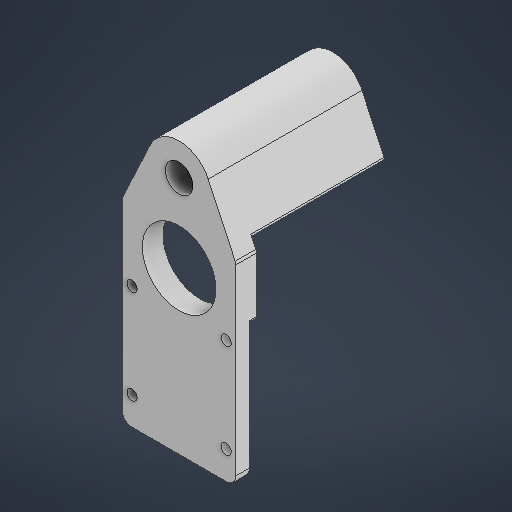
# Autodesk Inventor part: servo_side_plate1
Saved by Autodesk Inventor 2026 (Build 300175000, 175)
## iProperties
Created: 2025-12-05
Part Number: servo_side_plate1
Material: Generic
Document SubType Name: Modeling
Designer: numai
Density: 1 g/cm^3
Appearance: Default
Author: numai
Autodesk Inventor part; units mm, degrees
ref_plane "YZ Plane" through (0, 0, 0) normal (1, 0, 0) x (0, 1, 0)
ref_plane "XZ Plane" through (0, 0, 0) normal (0, 1, 0) x (-1, 0, 0)
ref_plane "XY Plane" through (0, 0, 0) normal (0, 0, 1) x (1, 0, 0)
ref_plane "作業平面1" through (0, -9.51851, 2.5) normal (0, 0, 1) x (1, 0, 0)
sketch "スケッチ1" plane through (0, -9.51851, 2.5) normal (0, 0, 1) x (1, 0, 0)
  arc A0 (6.110987, 12.224368) -> (9.975635, 16.20851) centre (0, 22.01851) ccw construction
  arc A1 (7, 11.230546) -> (6.110987, 12.224368) centre (6, 11.230546) ccw construction
  line L0 (7, 11.230546) -> (7, -12.09149) construction
  arc A2 (6.605696, -12.887186) -> (7, -12.09149) centre (6, -12.09149) ccw construction
  arc A3 (6.605696, -12.887186) -> (7.8, -11.59149) centre (6.5, -11.59149) ccw construction
  line L1 (7.8, -10.59149) -> (7.8, -11.59149) construction
  arc A4 (10.11, -8.28149) -> (7.8, -10.59149) centre (10.11, -10.59149) ccw construction
  line L2 (10.86, -8.28149) -> (10.11, -8.28149) construction
  arc A5 (10.86, -8.28149) -> (12.16, -6.98149) centre (10.86, -6.98149) ccw construction
  line L3 (12.16, 16.20851) -> (12.16, -6.98149) construction
  line L4 (9.975635, 16.20851) -> (12.16, 16.20851) construction
  circle A6 centre (10.25, 13.51851) radius 0.7835 construction
  circle A7 centre (10.25, -6.98149) radius 0.7835 construction
  arc A8 (-7.8, -11.59149) -> (-6.605696, -12.887186) centre (-6.5, -11.59149) ccw construction
  arc A9 (-7, -12.09149) -> (-6.605696, -12.887186) centre (-6, -12.09149) ccw construction
  line L5 (-7, -12.09149) -> (-7, 11.230546) construction
  arc A10 (-6.110987, 12.224368) -> (-7, 11.230546) centre (-6, 11.230546) ccw construction
  arc A11 (-9.975635, 16.20851) -> (-6.110987, 12.224368) centre (0, 22.01851) ccw construction
  line L6 (-12.16, 16.20851) -> (-9.975635, 16.20851) construction
  line L7 (-12.16, -6.98149) -> (-12.16, 16.20851) construction
  arc A12 (-12.16, -6.98149) -> (-10.86, -8.28149) centre (-10.86, -6.98149) ccw construction
  line L8 (-10.11, -8.28149) -> (-10.86, -8.28149) construction
  arc A13 (-7.8, -10.59149) -> (-10.11, -8.28149) centre (-10.11, -10.59149) ccw construction
  line L9 (-7.8, -11.59149) -> (-7.8, -10.59149) construction
  circle A14 centre (-10.25, 13.51851) radius 0.7835 construction
  circle A15 centre (-10.25, -6.98149) radius 0.7835 construction
  line L10 (-12.36, 16.20851) -> (-12.36, -6.98149) construction
  line L11 (12.36, -6.98149) -> (12.36, 16.20851) construction
  circle A16 centre (0, 22.01851) radius 3.4 construction
  arc A17 (5.25, 16.662439) -> (-5.25, 16.662439) centre (0, 22.01851) ccw construction
  arc A18 (-5.25, 16.662439) -> (5.25, 16.662439) centre (0, 22.01851) ccw construction
  circle A19 centre (0, 22.01851) radius 8
  arc A20 (10.25, -13.09149) -> (12.36, -10.98149) centre (10.25, -10.98149) ccw construction
  arc A21 (-12.36, -10.98149) -> (-10.25, -13.09149) centre (-10.25, -10.98149) ccw construction
  arc A22 (-11.92066, 29.86785) -> (-12.36, 28.80719) centre (-10.86, 28.80719) ccw
  line L12 (-10.09934, 31.689171) -> (-11.92066, 29.86785)
  arc A23 (-9.03868, 32.12851) -> (-10.09934, 31.689171) centre (-9.03868, 30.62851) ccw
  arc A24 (10.09934, 31.689171) -> (9.03868, 32.12851) centre (9.03868, 30.62851) ccw
  line L13 (11.92066, 29.86785) -> (10.09934, 31.689171)
  arc A25 (12.36, 28.80719) -> (11.92066, 29.86785) centre (10.86, 28.80719) ccw
  circle A26 centre (9.36, 29.12851) radius 0.7835 construction
  circle A27 centre (-9.36, 29.12851) radius 0.7835 construction
  line L14 (12.16, 16.40851) -> (9.975635, 16.40851) construction
  arc A28 (5.513943, 12.104473) -> (9.802811, 16.309167) centre (0, 22.01851) ccw construction
  arc A29 (-9.802811, 16.309167) -> (-5.513943, 12.104473) centre (0, 22.01851) ccw construction
  line L15 (-9.975635, 16.40851) -> (-12.16, 16.40851) construction
  line L16 (-12.36, 28.80719) -> (-12.36, 16.20851)
  line L17 (12.36, 16.20851) -> (12.36, 28.80719)
  line L18 (9.03868, 32.12851) -> (-9.03868, 32.12851)
  line L19 (12.36, 16.40851) -> (9.86, 16.40851)
  arc A30 (-9.86, 16.40851) -> (9.86, 16.40851) centre (0, 22.01851) ccw
  line L20 (-9.86, 16.40851) -> (-12.36, 16.40851)
  point P0 (0, 9.51851)
  dimension "d0" = 16
  constraints: 5 point on line, 4 end point, 2 centre point, 2 coincident, 2 point on circle, 1 concentric, 1 horizontal
  measures "d0" diameter of A19
extrude "押し出し1" add sketch "スケッチ1" against normal blind 2.5
sketch "スケッチ2" plane through (0, -9.51851, 2.5) normal (0, 0, 1) x (1, 0, 0)
  line L0 (-12.36, 28.80719) -> (-12.36, 16.40851)
  line L1 (-12.36, 16.40851) -> (-9.86, 16.40851)
  arc A0 (-9.86, 16.40851) -> (9.86, 16.40851) centre (0, 22.01851) ccw
  line L2 (9.86, 16.40851) -> (12.36, 16.40851)
  line L3 (12.36, 16.40851) -> (12.36, 28.80719)
  arc A1 (12.36, 28.80719) -> (11.92066, 29.86785) centre (10.86, 28.80719) ccw
  line L4 (11.92066, 29.86785) -> (10.09934, 31.689171)
  arc A2 (10.09934, 31.689171) -> (9.03868, 32.12851) centre (9.03868, 30.62851) ccw
  line L5 (9.03868, 32.12851) -> (-9.03868, 32.12851)
  arc A3 (-9.03868, 32.12851) -> (-10.09934, 31.689171) centre (-9.03868, 30.62851) ccw
  line L6 (-10.09934, 31.689171) -> (-11.92066, 29.86785)
  arc A4 (-11.92066, 29.86785) -> (-12.36, 28.80719) centre (-10.86, 28.80719) ccw
  circle A5 centre (0, 22.01851) radius 8
  line L7 (12.36, -10.98149) -> (12.36, -6.98149)
  line L8 (12.36, -6.98149) -> (12.36, 16.20851)
  line L9 (12.36, 16.20851) -> (12.36, 28.80719)
  line L10 (7, -12.09149) -> (7, 11.230546)
  arc A6 (10.25, -13.09149) -> (12.36, -10.98149) centre (10.25, -10.98149) ccw
  line L11 (6.5, -13.09149) -> (10.25, -13.09149)
  line L12 (-10.25, -13.09149) -> (-6.5, -13.09149)
  arc A7 (-12.36, -10.98149) -> (-10.25, -13.09149) centre (-10.25, -10.98149) ccw
  line L13 (-12.36, -6.98149) -> (-12.36, -10.98149)
  line L14 (-12.36, 16.20851) -> (-12.36, -6.98149)
  circle A8 centre (10.25, 13.51851) radius 0.7835 construction
  circle A9 centre (10.25, -6.98149) radius 0.7835 construction
  circle A10 centre (-10.25, 13.51851) radius 0.7835 construction
  circle A11 centre (-10.25, -6.98149) radius 0.7835 construction
  line L15 (-12.36, 28.80719) -> (-12.36, 16.20851)
  line L16 (-7, 11.230546) -> (-7, -12.09149)
  line L17 (7, 11.230546) -> (7, 13.09149)
  line L18 (7, -12.09149) -> (7, -13.09149)
  line L19 (-7, 11.230546) -> (-7, 13.09149)
  line L20 (-7, -12.09149) -> (-7, -13.09149)
  circle A12 centre (10.25, 13.51851) radius 1.1
  circle A13 centre (10.25, -6.98149) radius 1.1
  circle A14 centre (-10.25, 13.51851) radius 1.1
  circle A15 centre (-10.25, -6.98149) radius 1.1
  point P0 (0, 9.51851)
  dimension "d3" = 2.2
  constraints: 8 end point, 4 centre point, 4 coincident, 4 point on line, 3 equal radius, 2 point on circle, 1 parallel, 1 vertical
  measures "d3" diameter of A12
extrude "押し出し2" add sketch "スケッチ2" against normal blind 1 contours L1 A0 L19 L16 L20 L12 A7 L13 L14 L15 | A0 L2 L9 L8 L7 A6 L11 L18 L10 L17
sketch "スケッチ3" plane through (0, -9.51851, 2.5) normal (0, 0, 1) x (1, 0, 0)
  circle A0 centre (-10.25, 13.51851) radius 1.1
  circle A1 centre (-10.25, -6.98149) radius 1.1
  circle A2 centre (10.25, 13.51851) radius 1.1
  circle A3 centre (10.25, -6.98149) radius 1.1
  line L0 (-12.36, 28.80719) -> (-12.36, -10.98149)
  arc A4 (-12.36, -10.98149) -> (-10.25, -13.09149) centre (-10.25, -10.98149) ccw
  line L1 (-10.25, -13.09149) -> (-7, -13.09149)
  line L2 (-7, -13.09149) -> (-7, 13.09149)
  arc A5 (-7, 13.09149) -> (7, 13.09149) centre (0, 22.01851) ccw
  line L3 (7, 13.09149) -> (7, -13.09149)
  line L4 (7, -13.09149) -> (10.25, -13.09149)
  arc A6 (10.25, -13.09149) -> (12.36, -10.98149) centre (10.25, -10.98149) ccw
  line L5 (12.36, -10.98149) -> (12.36, 28.80719)
  arc A7 (12.36, 28.80719) -> (11.92066, 29.86785) centre (10.86, 28.80719) ccw
  line L6 (11.92066, 29.86785) -> (10.09934, 31.689171)
  arc A8 (10.09934, 31.689171) -> (9.03868, 32.12851) centre (9.03868, 30.62851) ccw
  line L7 (9.03868, 32.12851) -> (-9.03868, 32.12851)
  arc A9 (-9.03868, 32.12851) -> (-10.09934, 31.689171) centre (-9.03868, 30.62851) ccw
  line L8 (-10.09934, 31.689171) -> (-11.92066, 29.86785)
  arc A10 (-11.92066, 29.86785) -> (-12.36, 28.80719) centre (-10.86, 28.80719) ccw
  circle A11 centre (0, 22.01851) radius 8
  line L9 (7, -13.09149) -> (-7, -13.09149)
  point P0 (0, 9.51851)
  constraints: 2 end point, 1 collinear
extrude "押し出し3" add sketch "スケッチ3" along normal blind 2
sketch "スケッチ4" plane through (0, -9.51851, 4.5) normal (0, 0, 1) x (1, 0, 0)
  arc A0 (10.25, -13.09149) -> (12.36, -10.98149) centre (10.25, -10.98149) ccw
  line L0 (12.36, -10.98149) -> (12.36, 28.80719)
  arc A1 (12.36, 28.80719) -> (11.92066, 29.86785) centre (10.86, 28.80719) ccw
  line L1 (11.92066, 29.86785) -> (10.09934, 31.689171)
  arc A2 (10.09934, 31.689171) -> (9.03868, 32.12851) centre (9.03868, 30.62851) ccw
  line L2 (9.03868, 32.12851) -> (-9.03868, 32.12851)
  arc A3 (-9.03868, 32.12851) -> (-10.09934, 31.689171) centre (-9.03868, 30.62851) ccw
  line L3 (-10.09934, 31.689171) -> (-11.92066, 29.86785)
  arc A4 (-11.92066, 29.86785) -> (-12.36, 28.80719) centre (-10.86, 28.80719) ccw
  line L4 (-12.36, 28.80719) -> (-12.36, -10.98149)
  arc A5 (-12.36, -10.98149) -> (-10.25, -13.09149) centre (-10.25, -10.98149) ccw
  line L5 (-10.25, -13.09149) -> (10.25, -13.09149)
  circle A6 centre (-10.25, 13.51851) radius 1.1
  circle A7 centre (-10.25, -6.98149) radius 1.1
  circle A8 centre (10.25, 13.51851) radius 1.1
  circle A9 centre (10.25, -6.98149) radius 1.1
  circle A10 centre (0, 22.01851) radius 8
  line L6 (0, 22.01851) -> (0, 39.01851) construction
  circle A11 centre (0, 39.01851) radius 3
  circle A12 centre (0, 39.01851) radius 7 construction
  line L7 (-12.218223, 29.443768) -> (-6.338373, 41.989206)
  line L8 (12.218223, 29.443768) -> (6.338373, 41.989206)
  arc A13 (12.36, 28.80719) -> (11.92066, 29.86785) centre (10.86, 28.80719) ccw
  arc A14 (6.338373, 41.989206) -> (-6.338373, 41.989206) centre (0, 39.01851) ccw
  point P0 (0, 9.51851)
  dimension "d8" = 17
  dimension "d9" = 6
  dimension "d10" = 14
  constraints: 6 end point, 6 point on circle, 5 tangent, 3 centre point, 3 coincident, 1 vertical
  measures "d8" distance of L6.start L6.end
  measures "d9" diameter of A11
  measures "d10" diameter of A12
extrude "押し出し4" add sketch "スケッチ4" against normal up to surface (4.5 mm away) contours A1 L1 A2 L2 A3 L3 A4 L7 A14 L8
sketch "スケッチ5" plane through (0, -9.51851, 0) normal (0, 0, -1) x (-1, 0, 0)
  circle A0 centre (0, 39.01851) radius 3
  line L0 (12.36, 16.40851) -> (12.36, 28.80719)
  arc A1 (12.36, 28.80719) -> (12.218223, 29.443768) centre (10.86, 28.80719) ccw
  line L1 (12.218223, 29.443768) -> (6.338373, 41.989206)
  arc A2 (6.338373, 41.989206) -> (-6.338373, 41.989206) centre (0, 39.01851) ccw
  line L2 (-6.338373, 41.989206) -> (-12.218223, 29.443768)
  arc A3 (-12.218223, 29.443768) -> (-12.36, 28.80719) centre (-10.86, 28.80719) ccw
  line L3 (-12.36, 28.80719) -> (-12.36, 16.40851)
  line L4 (-12.36, 16.40851) -> (-9.86, 16.40851)
  arc A4 (-9.86, 16.40851) -> (9.86, 16.40851) centre (0, 22.01851) ccw
  line L5 (9.86, 16.40851) -> (12.36, 16.40851)
  circle A5 centre (0, 22.01851) radius 8
  arc A6 (-11.92066, 29.86785) -> (-12.36, 28.80719) centre (-10.86, 28.80719) ccw
  line L6 (-10.09934, 31.689171) -> (-11.92066, 29.86785)
  arc A7 (-9.03868, 32.12851) -> (-10.09934, 31.689171) centre (-9.03868, 30.62851) ccw
  line L7 (-0.95, 32.12851) -> (-9.03868, 32.12851)
  arc A8 (10.09934, 31.689171) -> (9.03868, 32.12851) centre (9.03868, 30.62851) ccw
  line L8 (11.92066, 29.86785) -> (10.09934, 31.689171)
  arc A9 (12.36, 28.80719) -> (11.92066, 29.86785) centre (10.86, 28.80719) ccw
  line L9 (9.03868, 32.12851) -> (0.95, 32.12851)
  line L10 (0.95, 32.12851) -> (-0.95, 32.12851)
  point P0 (0, 9.51851)
extrude "押し出し5" add sketch "スケッチ5" along normal blind 29 contours A9 L8 A8 L9 L10 L7 A7 L6 A6 L2 A2 L1
fillet "フィレット1" radius 0.4 2 edges at (12.2182, 19.9253, -14.5) (-12.2182, 19.9253, -14.5)
fillet "フィレット2" radius 0.4 4 edges at (7, -22.61, 2) (-7, -22.61, 2) (12.36, 6.89, 0.75) (-12.36, 6.89, 0.75)
sketch "スケッチ6" plane through (0, -9.51851, -29) normal (0, 0, -1) x (-1, 0, 0)
  circle A0 centre (0, 39.01851) radius 3
  circle A1 centre (0, 39.01851) radius 5
  point P0 (0, 9.51851)
  dimension "d17" = 10
  constraints: 1 centre point, 1 coincident
  measures "d17" diameter of A1
extrude "押し出し6" cut sketch "スケッチ6" against normal blind 1
